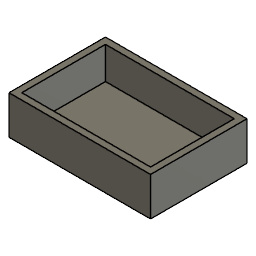
Sensor Housing (Autodesk Fusion 360 design; units mm, degrees)
part number: 2026-05-04-14-15-47-298
Autodesk Fusion 360 part; units mm, degrees
sketch "Sketch8" plane through (0, 0, 0) normal (0, 1, 0) x (-1, 0, 0)
  line L0 (0, 15) -> (22, 15)
  line L1 (22, 15) -> (22, 0)
  line L2 (22, 0) -> (0, 0)
  line L3 (0, 0) -> (0, 15)
  dimension "d23" = 22
  dimension "d24" = 15
  constraint horizontal L0
  constraint vertical L1
  constraint horizontal L2
  constraint vertical L3
  constraint coincident L2.end L3.start
  measures "d23" distance of L0.start L0.end
  measures "d24" distance of L0.start L2.end
extrude "Extrude5" add sketch "Sketch8" along normal blind 6
shell "Shell1" thickness 1 removed faces 1 at (-7.3333, 6, 10)
sketch "Sketch9" plane through (0, 1, 0) normal (0, 1, 0) x (-1, 0, 0)
  line L0 (1, 1) -> (21, 1)
  line L1 (21, 1) -> (21, 14)
  line L2 (21, 14) -> (1, 14)
  line L3 (1, 14) -> (1, 1)
  line L4 (4.712, 2) -> (2.112, 2)
  line L5 (2.112, 2) -> (2.112, 13.5)
  line L6 (2.112, 13.5) -> (4.712, 13.5)
  line L7 (4.712, 13.5) -> (4.712, 2)
  dimension "d28" = 2.6
  dimension "d29" = 11.5
  constraint horizontal L4
  constraint vertical L5
  constraint horizontal L6
  constraint vertical L7
  measures "d28" distance of L5 L7
  measures "d29" distance of L4.start L6.end
extrude "Extrude6" cut sketch "Sketch9" against normal blind 1.414 contours L4 L5 L6 L7
